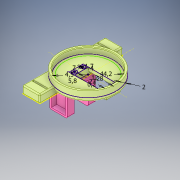
# Autodesk Inventor part: Mouth-Base
Saved by Autodesk Inventor 2018.3 (Build 223284000, 284)
## iProperties
Created: 2018-05-16
Part Number: Mouth-Base
Material: Generisch
Document SubType Name: Modeling
Designer: JochenAlt
Density: 1 g/cm^3
Appearance: Vorgabe
Author: JochenAlt
Autodesk Inventor part; units mm, degrees
ref_plane "YZ Plane" through (0, 0, 0) normal (1, 0, 0) x (0, 1, 0)
ref_plane "XZ Plane" through (0, 0, 0) normal (0, 1, 0) x (-1, 0, 0)
ref_plane "XY Plane" through (0, 0, 0) normal (0, 0, 1) x (1, 0, 0)
sketch "Skizze1" plane through (0, 0, 0) normal (0, 0, 1) x (1, 0, 0)
  circle A0 centre (0, 0) radius 22.1
  line L0 (0, 40.2232) -> (0, -36.7234) construction
  line L1 (-33.74, 0) -> (33.74, 0) construction
  circle A1 centre (0, 0) radius 24.1
  line L2 (-5.8, -6) -> (17.2, -6)
  line L3 (17.2, -6) -> (17.2, 6)
  line L4 (17.2, 6) -> (-5.8, 6)
  line L5 (-5.8, 6) -> (-5.8, -6)
  line L6 (-5.8, -6) -> (-10.3, -6)
  line L7 (-10.3, -6) -> (-10.3, 6)
  line L8 (-10.3, 6) -> (-5.8, 6)
  line L9 (-8.3, -3.5) -> (-8.3, 3.5) construction
  circle A2 centre (-8.3, -3.5) radius 0.85
  circle A3 centre (-8.3, 3.5) radius 0.85
  line L10 (17.2, -6) -> (21.7, -6)
  line L11 (21.7, -6) -> (21.7, 6)
  line L12 (21.7, 6) -> (17.2, 6)
  line L13 (19.7, -3.5) -> (19.7, 3.5) construction
  circle A4 centre (19.7, -3.5) radius 0.85
  circle A5 centre (19.7, 3.5) radius 0.85
  line L14 (5.7, -6) -> (5.7, 6) construction
  circle A6 centre (-8.3, 3.5) radius 2
  circle A7 centre (-8.3, -3.5) radius 2
  circle A8 centre (19.7, 3.5) radius 2
  circle A9 centre (19.7, -3.5) radius 2
  arc A10 (19.1836, 6) -> (19.1836, -6) centre (0, 0) ccw
  line L15 (-11.5375, -6.2) -> (0.4625, -6.2)
  dimension "d0" = 44.2
  dimension "d2" = 2
  dimension "d11" = 5.8
  dimension "d12" = 23
  dimension "d13" = 12
  dimension "d14" = 4.5
  dimension "d16" = 7
  dimension "d21" = 28
  dimension "d22" = 1.7
  dimension "d23" = 4
  dimension "d57" = 0.2
  constraints: 28 end point, 11 centre point, 10 coincident, 6 equal radius, 5 perpendicular, 4 horizontal, 2 equal length, 2 midpoint, 2 parallel, 2 point on circle, 2 point on line, 2 vertical, 1 symmetric about line, 2 other
  measures "d0" diameter of A0
  measures "d2" radial gap between concentric circles of A1 A0
  measures "d11" distance between parallel lines of L0 L5
  measures "d12" distance between parallel lines of L3 L5
  measures "d13" distance between parallel lines of L4 L2
  measures "d14" distance between parallel lines of L5 L7
  measures "d16" distance of L9.start L9.end
  measures "d21" distance between parallel lines of L13 L9
  measures "d22" diameter of A3
  measures "d23" diameter of A6
  measures "d57" distance between parallel lines of L2 L15
sketch "Skizze5" plane through (0, 0, 0) normal (0, 0, 1) x (1, 0, 0)
  line L0 (0, 40.2232) -> (0, -36.7234) construction
  line L1 (-20.9523, 0) -> (3.492, 0) construction
  line L2 (-19.3, 27.3) -> (-7.3, 27.3)
  line L3 (-7.3, 27.3) -> (-7.3, 7.5)
  line L4 (-7.3, 7.5) -> (-19.3, 7.5)
  line L5 (-19.3, 7.5) -> (-19.3, 27.3)
  line L6 (-19.3, -7.5) -> (-7.3, -7.5)
  line L7 (-7.3, -7.5) -> (-7.3, -27.3)
  line L8 (-7.3, -27.3) -> (-19.3, -27.3)
  line L9 (-19.3, -27.3) -> (-19.3, -7.5)
  line L10 (-5.8, -6) -> (-5.8, -35.8)
  line L11 (-20.8, -33.6077) -> (-20.8, -6)
  line L12 (-20.8, 6) -> (-20.8, 24.1569)
  line L13 (-19.3, 28.8) -> (-7.3, 28.8)
  line L14 (-5.8, 35.8) -> (-20.8, 35.8)
  line L15 (-20.8, 35.8) -> (-20.8, 26.3493)
  line L16 (-19.3, 27.3) -> (-19.3, 28.8)
  line L17 (-7.3, 27.3) -> (-7.3, 28.8)
  line L18 (-20.8, 24.1569) -> (-20.8, 26.3493)
  line L19 (-5.8, 6) -> (-5.8, 35.8)
  line L20 (-20.8, -35.8) -> (-5.8, -35.8)
  line L21 (-7.3, -28.8) -> (-19.3, -28.8)
  line L22 (-20.8, -35.8) -> (-20.8, -33.6077)
  line L23 (-19.3, -27.3) -> (-19.3, -28.8)
  line L24 (-7.3, -27.3) -> (-7.3, -28.8)
  line L25 (-20.8, 6) -> (-5.8, 6)
  line L26 (-20.8, -6) -> (-5.8, -6)
  line L27 (-7.3, -28.8) -> (-7.3, -34.3)
  line L28 (-19.3, -28.8) -> (-19.3, -34.3)
  line L29 (-7.3, 28.8) -> (-7.3, 34.3)
  line L30 (-19.3, 28.8) -> (-19.3, 34.3)
  line L31 (-7.3, -34.3) -> (-19.3, -34.3)
  line L32 (-7.3, 34.3) -> (-19.3, 34.3)
  line L33 (-5.8, 6) -> (-5.8, -6) construction
  line L34 (-10.3, -6) -> (-10.3, 6) construction
  point P0 (0, 0)
  dimension "d60" = 12
  dimension "d66" = 1.5
  dimension "d67" = 1.5
  dimension "d69" = 1.5
  dimension "d70" = 1.5
  dimension "d72" = 19.8
  dimension "d73" = 1.5
  dimension "d74" = 1.5
  dimension "d83" = 5.5
  dimension "d84" = 1.5
  dimension "d85" = 5.5
  dimension "d86" = 1.5
  dimension "d87" = 6
  constraints: 62 end point, 9 vertical, 7 perpendicular, 6 parallel, 5 horizontal, 4 collinear, 3 equal length, 1 other
  measures "d60" distance of L2.start L2.end
  measures "d66" distance between parallel lines of L26 L6
  measures "d67" distance between parallel lines of L13 L2
  measures "d69" distance between parallel lines of L16 L18
  measures "d70" distance between parallel lines of L8 L21
  measures "d72" distance between parallel lines of L2 L4
  measures "d73" distance between parallel lines of L25 L4
  measures "d74" distance between parallel lines of L19 L3
  measures "d83" distance between parallel lines of L31 L21
  measures "d84" distance between parallel lines of L20 L31
  measures "d85" distance between parallel lines of L32 L13
  measures "d86" distance between parallel lines of L14 L32
  measures "d87" distance between parallel lines of L25 L1
extrude "Extrusion1" add sketch "Skizze1" along normal blind 5 contours A0 L12 L11 | L11 L10 A0 | A1
extrude "Extrusion2" add sketch "Skizze1" against normal blind 3 contours A0 L11 | A9 | A8 | L11 A0 L10 L3 L12 | A0 L12 L11 | L11 L10 A0 | L12 A10 L10 A0 | L12 L4 L8 L7 L6 L2 L10 A10 | A6 | A7 | L5 L6 L7 L8 | A1
chamfer "Fase1" distance 0.5 angle 45 1 edges at (-22.1, 0, 5)
extrude "Extrusion3" add sketch "Skizze1" against normal blind 2 from surface at -3 contours A9 | A8 | L11 A0 L10 L3 L12 | A0 L12 L11 | L11 L10 A0 | A6 | A7 | L5 L6 L7 L8
extrude "Extrusion4" cut sketch "Skizze1" against normal blind 2 contours A9 | A8 | A6 | A7 | A2 | A3 | A4 | A5
extrude "Extrusion10" add sketch "Skizze5" against normal blind 5 contours L2 L3 L4 L5 | L30 L32 L29 L13 | L6 L7 L8 L9 | L21 L27 L31 L28 | L10 L20 L22 L11 L26 | L12 L18 L15 L14 L19 L25
extrude "Extrusion12" add sketch "Skizze5" against normal blind 1 from surface at -5
ref_plane "Arbeitsebene1" through (-5.8, 6, -6.5) normal (0, 0, -1) x (-1, 0, 0)
sketch "Skizze7" plane through (0, 0, -6.5) normal (0, 0, 1) x (1, 0, 0)
  line L0 (-10.3, 6) -> (-5.8, 6) projected
  line L1 (-5.8, 6) -> (-5.8, -6) projected
  line L2 (-5.8, -6) -> (-10.3, -6) projected
  line L3 (-10.3, -6) -> (-10.3, 6) projected
  circle A0 centre (-8.3, -3.5) radius 0.85 projected
  circle A1 centre (-8.3, 3.5) radius 0.85 projected
  line L4 (-5.8, -35.8) -> (-20.8, -35.8) projected
  line L5 (-20.8, -35.8) -> (-20.8, -6) projected
  line L6 (-20.8, -6) -> (-5.8, -6) projected
  line L7 (-5.8, -6) -> (-5.8, -35.8) projected
  line L8 (-19.3, -34.3) -> (-7.3, -34.3) projected
  line L9 (-7.3, -34.3) -> (-7.3, -7.5) projected
  line L10 (-7.3, -7.5) -> (-19.3, -7.5) projected
  line L11 (-19.3, -7.5) -> (-19.3, -34.3) projected
  line L12 (-7.3, 34.3) -> (-19.3, 34.3) projected
  line L13 (-19.3, 34.3) -> (-19.3, 7.5) projected
  line L14 (-19.3, 7.5) -> (-7.3, 7.5) projected
  line L15 (-7.3, 7.5) -> (-7.3, 34.3) projected
  line L16 (-5.8, 6) -> (-20.8, 6) projected
  line L17 (-20.8, 6) -> (-20.8, 35.8) projected
  line L18 (-20.8, 35.8) -> (-5.8, 35.8) projected
  line L19 (-5.8, 35.8) -> (-5.8, 6) projected
  line L20 (-20.8, -6) -> (-20.8, -12.1725) projected
  line L21 (-20.8, 6) -> (-20.8, 35.8) projected
  line L22 (-5.8, 12.1725) -> (-7.3, 12.1725)
  line L23 (-19.3, 12.1725) -> (-20.8, 12.1725)
  line L24 (-5.8, -12.1725) -> (-7.3, -12.1725)
  line L25 (-19.3, -12.1725) -> (-20.8, -12.1725)
  line L26 (-7.3, -12.1725) -> (-19.3, -12.1725)
  line L27 (-7.3, -34.3) -> (-7.3, -7.5) projected
  line L28 (-7.3, 12.1725) -> (-19.3, 12.1725)
  line L29 (-19.3, 7.5) -> (-19.3, 27.3) projected
  arc A2 (-20.8, 12.1725) -> (-20.8, -12.1725) centre (0, 0) ccw projected
  line L30 (-10.3, -6) -> (-10.3, 6) projected
  line L31 (-20.8, 12.1725) -> (-20.8, 6) projected
  line L32 (-20.8, 6) -> (-10.3, 6) projected
  line L33 (-10.3, 6) -> (-10.3, -6) projected
  line L34 (-10.3, -6) -> (-20.8, -6) projected
  line L35 (-20.8, -6) -> (-20.8, -12.1725) projected
  arc A3 (-20.8, 12.1725) -> (-20.8, -12.1725) centre (0, 0) ccw projected
  constraints: 12 end point, 7 point on line, 4 horizontal, 2 collinear, 2 perpendicular
extrude "Extrusion14" add sketch "Skizze7" against normal blind 3 separate body contours L16 L17 L23 L13 L14 L15 L22 L19 L0 | L0 L1 L2 L3 | L3 L6 L5 A2 L17 L16 | L2 L7 L24 L9 L10 L11 L25 L5 L6
extrude "Extrusion15" add sketch "Skizze7" along normal up to surface (0.5 mm away) contours L16 L17 L23 L13 L14 L15 L22 L19 L0 | L2 L7 L24 L9 L10 L11 L25 L5 L6 bodies 2
extrude "Extrusion16" add sketch "Skizze7" against normal blind 21.5 contours L16 L17 L23 L13 L14 L15 L22 L19 L0 | L2 L7 L24 L9 L10 L11 L25 L5 L6 bodies 2
extrude "Extrusion17" add sketch "Skizze7" against normal blind 1.5 from surface at -21.5 contours L16 L17 L23 L13 L14 L15 L22 L19 L0 | L2 L7 L24 L9 L10 L11 L25 L5 L6 | L15 L14 L13 L28 | L26 L11 L10 L9 bodies 2
extrude "Extrusion18" add sketch "Skizze7" along normal up to surface (3.5 mm away) contours L3 L6 L5 A2 L17 L16 bodies 2
fillet "Rundung3" radius 1 16 edges at (-20.8, 35.8, -2.5) (-20.8, 35.8, -5.5) (-5.8, 35.8, -2.5) (-5.8, 35.8, -5.5) (-20.8, -35.8, -2.5) (-20.8, -35.8, -5.5) (-5.8, -35.8, -2.5) (-5.8, -35.8, -5.5) (-20.8, -9.0863, -9.5) (-20.8, 9.0863, -9.5) (-13.3, 6, -9.5) (-13.3, -6, -9.5) (-20.8, 9.0863, -29.5) (-5.8, 9.0863, -29.5) (-20.8, -9.0863, -29.5) (-5.8, -9.0863, -29.5)
fillet "Rundung3" radius 1 8 edges at (14.8497, 18.9814, -3) (14.8497, -18.9814, -3) (-20.8, 23.9863, 0) (-13.3, 35.8, 0) (-5.8, 29.5958, 0) (-13.3, -35.8, 0) (-5.8, -29.5958, 0) (-20.8, -23.9863, 0)
equation "\"d70\" = d67"
equation "\"d64\" = d59"
equation "\"d59\" = 1"
